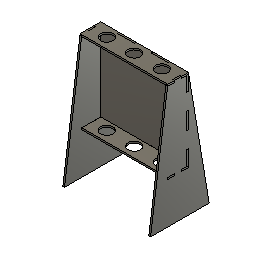
OpenColumnx3_FitSBS_v1 v6 (Autodesk Fusion 360 design; units mm, degrees)
Autodesk Fusion 360 part; units mm, degrees
sketch "Sketch1" plane through (0, 0, 0) normal (0, 1, 0) x (1, 0, 0)
  line L0 (0, 0) -> (127.76, 0)
  line L1 (127.76, 0) -> (127.76, 85.48)
  line L2 (127.76, 85.48) -> (0, 85.48)
  line L3 (0, 85.48) -> (0, 0)
  line L4 (0, 85.48) -> (2.5, 85.48)
  line L5 (2.5, 85.48) -> (2.5, 0)
  line L6 (2.5, 0) -> (0, 0)
  line L7 (0, 0) -> (0, 85.48)
  line L8 (127.76, 85.48) -> (125.26, 85.48)
  line L9 (125.26, 85.48) -> (125.26, 0)
  line L10 (125.26, 0) -> (127.76, 0)
  line L11 (127.76, 0) -> (127.76, 85.48)
  dimension "d1" = 127.76
  dimension "d2" = 85.48
  dimension "d3" = 2.5
  dimension "d4" = 85.48
  dimension "d5" = 2.5
  constraint horizontal L0
  constraint vertical L1
  constraint horizontal L2
  constraint vertical L3
  constraint coincident L0.start L3.end
  constraint horizontal L4
  constraint vertical L5
  constraint horizontal L6
  constraint vertical L7
  constraint horizontal L8
  constraint vertical L9
  constraint horizontal L10
  constraint vertical L11
  constraint coincident L0 L9.end
  measures "d1" distance of L0.start L0.end
  measures "d2" distance of L0.start L2.end
  measures "d3" distance of L2.end L4.end
  measures "d4" distance of L2.end L0.start
  measures "d5" distance of L1.end L8.end
ref_plane "WorkPlane1" through (0, 45, 0) normal (0, 1, 0) x (0, 0, 1)
ref_plane "WorkPlane2" through (0, 60, 0) normal (0, 1, 0) x (0, 0, 1)
sketch "Sketch2" plane through (0, 60, 0) normal (0, 1, 0) x (1, 0, 0)
  line L0 (0, 0) -> (127.76, 0)
  line L1 (127.76, 0) -> (127.76, 85.48)
  line L2 (127.76, 85.48) -> (0, 85.48)
  line L3 (0, 85.48) -> (0, 0)
  line L4 (127.76, 55.24) -> (0, 55.24)
  line L5 (0, 55.24) -> (0, 25.24)
  line L6 (0, 25.24) -> (127.76, 25.24)
  line L7 (127.76, 25.24) -> (127.76, 55.24)
  line L8 (127.76, 55.24) -> (0, 25.24) construction
  line L9 (0, 55.24) -> (127.76, 25.24) construction
  line L10 (0, 25.24) -> (2.5, 25.24)
  line L11 (2.5, 25.24) -> (2.5, 55.24)
  line L12 (2.5, 55.24) -> (0, 55.24)
  line L13 (0, 55.24) -> (0, 25.24)
  line L14 (127.76, 25.24) -> (125.26, 25.24)
  line L15 (125.26, 25.24) -> (125.26, 55.24)
  line L16 (125.26, 55.24) -> (127.76, 55.24)
  line L17 (127.76, 55.24) -> (127.76, 25.24)
  circle A0 centre (63.88, 40.24) radius 9
  circle A1 centre (63.88, 40.24) radius 18
  circle A2 centre (23.88, 40.24) radius 9
  circle A3 centre (23.88, 40.24) radius 18
  circle A4 centre (103.88, 40.24) radius 9
  circle A5 centre (103.88, 40.24) radius 18
  line L18 (127.76, 25.24) -> (125.26, 25.24)
  line L19 (0, 25.24) -> (2.5, 25.24)
  line L20 (0, 25.24) -> (2.5, 25.24)
  line L21 (127.76, 35.24) -> (125.26, 35.24)
  line L22 (0, 35.24) -> (2.5, 35.24)
  line L23 (127.76, 45.24) -> (125.26, 45.24)
  line L24 (0, 45.24) -> (2.5, 45.24)
  line L25 (127.76, 55.24) -> (125.26, 55.24)
  line L26 (0, 55.24) -> (2.5, 55.24)
  line L27 (0, 55.24) -> (127.76, 55.24)
  line L28 (127.76, 55.24) -> (127.76, 52.74)
  line L29 (127.76, 52.74) -> (0, 52.74)
  line L30 (0, 52.74) -> (0, 55.24)
  line L31 (2.5, 55.24) -> (2.5, 52.74)
  line L32 (27.052, 55.24) -> (27.052, 52.74)
  line L33 (51.604, 55.24) -> (51.604, 52.74)
  line L34 (76.156, 55.24) -> (76.156, 52.74)
  line L35 (100.708, 55.24) -> (100.708, 52.74)
  line L36 (125.26, 55.24) -> (125.26, 52.74)
  line L37 (2.5, 52.74) -> (0, 52.74)
  line L38 (0, 52.74) -> (0, 55.24)
  line L39 (0, 55.24) -> (2.5, 55.24)
  line L40 (2.5, 55.24) -> (2.5, 52.74)
  line L41 (125.26, 52.74) -> (127.76, 52.74)
  line L42 (127.76, 52.74) -> (127.76, 55.24)
  line L43 (127.76, 55.24) -> (125.26, 55.24)
  line L44 (125.26, 55.24) -> (125.26, 52.74)
  point P0 (63.88, 40.24)
  dimension "d8" = 127.76
  dimension "d9" = 85.48
  dimension "d10" = 127.76
  dimension "d11" = 30
  dimension "d12" = 2.5
  dimension "d13" = 2.5
  dimension "d14" = 18
  dimension "d15" = 36
  dimension "d18" = 40
  dimension "d19" = 0
  dimension "d33" = 0
  dimension "d34" = 30
  dimension "d37" = 2.5
  dimension "d40" = 122.76
  dimension "d41" = 0
  constraint horizontal L0
  constraint vertical L1
  constraint horizontal L2
  constraint vertical L3
  constraint coincident L0.start L3.end
  constraint horizontal L4
  constraint perpendicular L4 L5
  constraint parallel L4 L6
  constraint parallel L5 L7
  constraint coincident L8 P0
  constraint coincident L9 P0
  constraint horizontal L10
  constraint vertical L11
  constraint horizontal L12
  constraint vertical L13
  constraint coincident L4 L11.end
  constraint horizontal L14
  constraint vertical L15
  constraint horizontal L16
  constraint vertical L17
  constraint coincident L4 L15.end
  constraint coincident P0 A0.centre
  constraint concentric A0 A1
  constraint horizontal L27
  constraint vertical L28
  constraint horizontal L29
  constraint vertical L30
  constraint coincident L29 L31.end
  constraint coincident L11 L31.end
  constraint horizontal L37
  constraint vertical L38
  constraint horizontal L39
  constraint vertical L40
  constraint horizontal L41
  constraint vertical L42
  constraint horizontal L43
  constraint vertical L44
  measures "d8" distance of L0.start L0.end
  measures "d9" distance of L0.start L2.end
  measures "d10" distance of L5.end L6.end
  measures "d11" distance of L4.end L5.end
  measures "d12" distance of L5.end L10.end
  measures "d13" distance of L6.end L14.end
  measures "d14" diameter of A0
  measures "d15" diameter of A1
  measures "d37" distance of L4.end L29.end
extrude "Extrude3" add sketch "Sketch2" along normal blind 2.5 contours L3 L5 L6 L10 L11 L13 L19 L20 L22 | L1 L6 L7 L14 L15 L17 L18 L21 | L6 L11 A3 L29 | L6 L15 A5 L29 | L3 L5 L11 L13 L24 L29 L37 | L6 A3 L29 | L1 L7 L15 L17 L23 L29 L41 | L6 A5 L29 | L3 L4 L5 L11 L12 L13 L26 L27 L29 L30 L31 L37 L38 L39 L40 | L6 A1 A3 L29 | L4 L11 A3 L27 L29 L31 L40 | L4 A3 L27 L29 L32 | L1 L4 L7 L15 L16 L17 L25 L27 L28 L29 L36 L41 L42 L43 L44 | L6 A1 A5 L29 | L6 A1 L29 | L4 L15 A5 L27 L29 L36 L44 | L4 A5 L27 L29 L35 | L4 A1 L27 L33 | L4 A1 L27 L29 L33 L34 | L4 A1 L27 L34 picked at (22.678, 54.4067) picked at (105.082, 54.4067) makes body 1
copy_body "CopyPasteBodies3" bodies 1 makes body 2
move_body "Move3" bodies 2 to x (1, 0, 0) y (0, 1, 0) z (0, 0, 1) at (0, 117.5, 0)
sketch "Sketch4" plane through (0, 180, 0) normal (0, 1, 0) x (-1, 0, 0)
  circle A0 centre (-103.88, -40.24) radius 9
  circle A1 centre (-23.88, -40.24) radius 9
  circle A2 centre (-63.88, -40.24) radius 9
  line L0 (-127.76, -55.24) -> (-100.708, -55.24)
  line L1 (-100.708, -55.24) -> (-100.708, -52.74)
  line L2 (-100.708, -52.74) -> (-76.156, -52.74)
  line L3 (-76.156, -52.74) -> (-76.156, -55.24)
  line L4 (-76.156, -55.24) -> (-51.604, -55.24)
  line L5 (-51.604, -55.24) -> (-51.604, -52.74)
  line L6 (-51.604, -52.74) -> (-27.052, -52.74)
  line L7 (-27.052, -52.74) -> (-27.052, -55.24)
  line L8 (-27.052, -55.24) -> (0, -55.24)
  line L9 (0, -55.24) -> (0, -45.24)
  line L10 (0, -45.24) -> (-2.5, -45.24)
  line L11 (-2.5, -45.24) -> (-2.5, -35.24)
  line L12 (-2.5, -35.24) -> (0, -35.24)
  line L13 (0, -35.24) -> (0, -25.24)
  line L14 (0, -25.24) -> (-127.76, -25.24)
  line L15 (-127.76, -25.24) -> (-127.76, -35.24)
  line L16 (-127.76, -35.24) -> (-125.26, -35.24)
  line L17 (-125.26, -35.24) -> (-125.26, -45.24)
  line L18 (-125.26, -45.24) -> (-127.76, -45.24)
  line L19 (-127.76, -45.24) -> (-127.76, -55.24)
  line L20 (-127.76, -25.24) -> (-125.26, -25.24)
  line L21 (-125.26, -25.24) -> (-125.26, -55.24)
  line L22 (-125.26, -55.24) -> (-127.76, -55.24)
  line L23 (-127.76, -55.24) -> (-127.76, -25.24)
  line L24 (0, -25.24) -> (-2.5, -25.24)
  line L25 (-2.5, -25.24) -> (-2.5, -55.24)
  line L26 (-2.5, -55.24) -> (0, -55.24)
  line L27 (0, -55.24) -> (0, -25.24)
  dimension "d44" = 2.5
  dimension "d45" = 30
  dimension "d46" = 2.5
  dimension "d47" = 30
  constraint horizontal L20
  constraint vertical L21
  constraint horizontal L22
  constraint vertical L23
  constraint coincident L14.end L15.start
  constraint horizontal L24
  constraint vertical L25
  constraint horizontal L26
  constraint vertical L27
  constraint coincident L13.end L14.start
  measures "d44" distance of L14.end L20.end
  measures "d45" distance of L14.end L0.start
  measures "d46" distance of L13.end L24.end
  measures "d47" distance of L13.end L8.end
loft "Loft3" add profiles "Sketch4", "Sketch1" section 1 contours L0 L18 L19 L21 L22 L23 | L16 L17 L18 L21 L23 | L14 L15 L16 L20 L21 L23 section 2 contours L0 L1 L2 L8 L9 L10 L11 separate body makes body 3
loft "Loft4" add profiles "Sketch4", "Sketch1" section 1 contours L12 L13 L14 L24 L25 L27 | L10 L11 L12 L25 L27 | L8 L9 L10 L25 L26 L27 section 2 contours L0 L2 L3 L4 L5 L6 L7 separate body makes body 4
ref_plane "WorkPlane3" through (39.328, 178.75, -52.74) normal (0, 0, -1) x (-1, 0, 0)
extrude "Extrude4" add sketch "Sketch2" along normal blind 120 separate body contours L3 L4 L5 L11 L12 L13 L26 L27 L29 L30 L31 L37 L38 L39 L40 | L4 L11 A3 L27 L29 L31 L40 | L4 A3 L27 L29 L32 | L1 L4 L7 L15 L16 L17 L25 L27 L28 L29 L36 L41 L42 L43 L44 | L4 A3 L27 L29 L32 | L4 L15 A5 L27 L29 L36 L44 | L4 A1 A5 L27 L29 L34 | L4 A5 L27 L29 L35 | L4 A5 L27 L29 L35 | L4 A1 A3 L27 L29 L33 | A1 L29 L33 | A1 L29 L34 | L4 A1 L27 L33 | L4 A1 L27 L29 L33 L34 | L4 A1 L27 L34 makes body 5
sketch "Sketch7" plane through (0, 0, -55.24) normal (0, 0, -1) x (-1, 0, 0)
  line L0 (-127.76, 60) -> (0, 60)
  line L1 (0, 60) -> (0, 180)
  line L2 (0, 180) -> (-127.76, 180)
  line L3 (-127.76, 180) -> (-127.76, 60)
  line L4 (-127.76, 180) -> (0, 180)
  line L5 (0, 180) -> (0, 60)
  line L6 (0, 60) -> (-127.76, 60)
  line L7 (-127.76, 60) -> (-127.76, 180)
  line L8 (-127.76, 180) -> (-125.26, 180)
  line L9 (-125.26, 180) -> (-125.26, 60)
  line L10 (-125.26, 60) -> (-127.76, 60)
  line L11 (-127.76, 60) -> (-127.76, 180)
  line L12 (0, 180) -> (-2.5, 180)
  line L13 (-2.5, 180) -> (-2.5, 60)
  line L14 (-2.5, 60) -> (0, 60)
  line L15 (0, 60) -> (0, 180)
  line L16 (-127.76, 180) -> (-125.26, 180)
  line L17 (0, 180) -> (-2.5, 180)
  line L18 (0, 156) -> (-2.5, 156)
  line L19 (0, 132) -> (-2.5, 132)
  line L20 (0, 108) -> (-2.5, 108)
  line L21 (0, 84) -> (-2.5, 84)
  line L22 (0, 60) -> (-2.5, 60)
  line L23 (-127.76, 156) -> (-125.26, 156)
  line L24 (-127.76, 132) -> (-125.26, 132)
  line L25 (-127.76, 108) -> (-125.26, 108)
  line L26 (-127.76, 84) -> (-125.26, 84)
  line L27 (-127.76, 60) -> (-125.26, 60)
  dimension "d51" = 2.5
  dimension "d52" = 2.5
  dimension "d53" = 120
  dimension "d56" = 0
  dimension "d57" = -120
  dimension "d60" = 0
  dimension "d61" = -120
  constraint horizontal L4
  constraint vertical L5
  constraint horizontal L6
  constraint vertical L7
  constraint coincident L0.end L1.start
  constraint coincident L2.end L3.start
  constraint horizontal L8
  constraint vertical L9
  constraint horizontal L10
  constraint vertical L11
  constraint horizontal L12
  constraint vertical L13
  constraint horizontal L14
  constraint vertical L15
  measures "d51" distance of L2.end L8.end
  measures "d52" distance of L1.end L12.end
  measures "d53" distance of L1.end L0.end
extrude "Extrude5" cut sketch "Sketch7" against normal blind 20 contours L3 L7 L9 L11 L25 L26 | L1 L5 L13 L15 L20 L21 | L3 L7 L9 L11 L23 L24 | L1 L5 L13 L15 L18 L19 bodies 5
combine "Combine1" operation cut target body 5 tool bodies 2 1 keep tools
combine "Combine2" operation cut target body 4 tool bodies 2 5 1 keep tools
combine "Combine3" operation cut target body 3 tool bodies 5 2 1 keep tools
sketch "Sketch8" plane through (127.76, 0, 0) normal (1, 0, 0) x (0, 0, -1)
  line L0 (45.24, 62.5) -> (52.74, 62.5)
  line L1 (52.74, 62.5) -> (52.74, 84)
  line L2 (52.74, 84) -> (55.24, 84)
  line L3 (55.24, 84) -> (55.24, 60)
  line L4 (55.24, 60) -> (45.24, 60)
  line L5 (45.24, 60) -> (45.24, 62.5)
  line L6 (25.24, 60) -> (25.24, 62.5)
  line L7 (25.24, 62.5) -> (35.24, 62.5)
  line L8 (35.24, 62.5) -> (35.24, 60)
  line L9 (35.24, 60) -> (25.24, 60)
  line L10 (25.24, 177.5) -> (25.24, 180)
  line L11 (25.24, 180) -> (0, 0)
  line L12 (0, 0) -> (85.48, 0)
  line L13 (85.48, 0) -> (55.24, 180)
  line L14 (55.24, 180) -> (55.24, 156)
  line L15 (55.24, 156) -> (52.74, 156)
  line L16 (52.74, 156) -> (52.74, 177.5)
  line L17 (52.74, 177.5) -> (45.24, 177.5)
  line L18 (45.24, 177.5) -> (45.24, 180)
  line L19 (45.24, 180) -> (35.24, 180)
  line L20 (35.24, 180) -> (35.24, 177.5)
  line L21 (35.24, 177.5) -> (25.24, 177.5)
  line L22 (55.24, 132) -> (55.24, 108)
  line L23 (55.24, 108) -> (52.74, 108)
  line L24 (52.74, 108) -> (52.74, 132)
  line L25 (52.74, 132) -> (55.24, 132)
sketch "Sketch9" plane through (0, 0, -52.74) normal (0, 0, 1) x (1, 0, 0)
  line L0 (0, 62.5) -> (27.052, 62.5)
  line L1 (27.052, 62.5) -> (27.052, 60)
  line L2 (27.052, 60) -> (51.604, 60)
  line L3 (51.604, 60) -> (51.604, 62.5)
  line L4 (51.604, 62.5) -> (76.156, 62.5)
  line L5 (76.156, 62.5) -> (76.156, 60)
  line L6 (76.156, 60) -> (100.708, 60)
  line L7 (100.708, 60) -> (100.708, 62.5)
  line L8 (100.708, 62.5) -> (127.76, 62.5)
  line L9 (127.76, 62.5) -> (127.76, 84)
  line L10 (127.76, 84) -> (125.26, 84)
  line L11 (125.26, 84) -> (125.26, 108)
  line L12 (125.26, 108) -> (127.76, 108)
  line L13 (127.76, 108) -> (127.76, 132)
  line L14 (127.76, 132) -> (125.26, 132)
  line L15 (125.26, 132) -> (125.26, 156)
  line L16 (125.26, 156) -> (127.76, 156)
  line L17 (127.76, 156) -> (127.76, 177.5)
  line L18 (127.76, 177.5) -> (100.708, 177.5)
  line L19 (100.708, 177.5) -> (100.708, 180)
  line L20 (100.708, 180) -> (76.156, 180)
  line L21 (76.156, 180) -> (76.156, 177.5)
  line L22 (76.156, 177.5) -> (51.604, 177.5)
  line L23 (51.604, 177.5) -> (51.604, 180)
  line L24 (51.604, 180) -> (27.052, 180)
  line L25 (27.052, 180) -> (27.052, 177.5)
  line L26 (27.052, 177.5) -> (0, 177.5)
  line L27 (0, 177.5) -> (0, 156)
  line L28 (0, 156) -> (2.5, 156)
  line L29 (2.5, 156) -> (2.5, 132)
  line L30 (2.5, 132) -> (0, 132)
  line L31 (0, 132) -> (0, 108)
  line L32 (0, 108) -> (2.5, 108)
  line L33 (2.5, 108) -> (2.5, 84)
  line L34 (2.5, 84) -> (0, 84)
  line L35 (0, 84) -> (0, 62.5)
sketch "Sketch10" plane through (0, 180, 0) normal (0, 1, 0) x (-1, 0, 0)
  circle A0 centre (-103.88, -40.24) radius 9
  circle A1 centre (-23.88, -40.24) radius 9
  circle A2 centre (-63.88, -40.24) radius 9
  line L0 (-127.76, -55.24) -> (-100.708, -55.24)
  line L1 (-100.708, -55.24) -> (-100.708, -52.74)
  line L2 (-100.708, -52.74) -> (-76.156, -52.74)
  line L3 (-76.156, -52.74) -> (-76.156, -55.24)
  line L4 (-76.156, -55.24) -> (-51.604, -55.24)
  line L5 (-51.604, -55.24) -> (-51.604, -52.74)
  line L6 (-51.604, -52.74) -> (-27.052, -52.74)
  line L7 (-27.052, -52.74) -> (-27.052, -55.24)
  line L8 (-27.052, -55.24) -> (0, -55.24)
  line L9 (0, -55.24) -> (0, -45.24)
  line L10 (0, -45.24) -> (-2.5, -45.24)
  line L11 (-2.5, -45.24) -> (-2.5, -35.24)
  line L12 (-2.5, -35.24) -> (0, -35.24)
  line L13 (0, -35.24) -> (0, -25.24)
  line L14 (0, -25.24) -> (-127.76, -25.24)
  line L15 (-127.76, -25.24) -> (-127.76, -35.24)
  line L16 (-127.76, -35.24) -> (-125.26, -35.24)
  line L17 (-125.26, -35.24) -> (-125.26, -45.24)
  line L18 (-125.26, -45.24) -> (-127.76, -45.24)
  line L19 (-127.76, -45.24) -> (-127.76, -55.24)
sketch "Sketch11" plane through (0, 0, 0) normal (-1, 0, 0) x (0, 0, 1)
  line L0 (-55.24, 60) -> (-55.24, 84)
  line L1 (-55.24, 84) -> (-52.74, 84)
  line L2 (-52.74, 84) -> (-52.74, 62.5)
  line L3 (-52.74, 62.5) -> (-45.24, 62.5)
  line L4 (-45.24, 62.5) -> (-45.24, 60)
  line L5 (-45.24, 60) -> (-55.24, 60)
  line L6 (-35.24, 60) -> (-35.24, 62.5)
  line L7 (-35.24, 62.5) -> (-25.24, 62.5)
  line L8 (-25.24, 62.5) -> (-25.24, 60)
  line L9 (-25.24, 60) -> (-35.24, 60)
  line L10 (-52.74, 177.5) -> (-52.74, 156)
  line L11 (-52.74, 156) -> (-55.24, 156)
  line L12 (-55.24, 156) -> (-55.24, 180)
  line L13 (-55.24, 180) -> (-85.48, 0)
  line L14 (-85.48, 0) -> (0, 0)
  line L15 (0, 0) -> (-25.24, 180)
  line L16 (-25.24, 180) -> (-25.24, 177.5)
  line L17 (-25.24, 177.5) -> (-35.24, 177.5)
  line L18 (-35.24, 177.5) -> (-35.24, 180)
  line L19 (-35.24, 180) -> (-45.24, 180)
  line L20 (-45.24, 180) -> (-45.24, 177.5)
  line L21 (-45.24, 177.5) -> (-52.74, 177.5)
  line L22 (-55.24, 108) -> (-55.24, 132)
  line L23 (-55.24, 132) -> (-52.74, 132)
  line L24 (-52.74, 132) -> (-52.74, 108)
  line L25 (-52.74, 108) -> (-55.24, 108)
sketch "Sketch12" plane through (0, 62.5, 0) normal (0, 1, 0) x (-1, 0, 0)
  circle A0 centre (-103.88, -40.24) radius 9
  circle A1 centre (-23.88, -40.24) radius 9
  circle A2 centre (-63.88, -40.24) radius 9
  line L0 (-127.76, -55.24) -> (-100.708, -55.24)
  line L1 (-100.708, -55.24) -> (-100.708, -52.74)
  line L2 (-100.708, -52.74) -> (-76.156, -52.74)
  line L3 (-76.156, -52.74) -> (-76.156, -55.24)
  line L4 (-76.156, -55.24) -> (-51.604, -55.24)
  line L5 (-51.604, -55.24) -> (-51.604, -52.74)
  line L6 (-51.604, -52.74) -> (-27.052, -52.74)
  line L7 (-27.052, -52.74) -> (-27.052, -55.24)
  line L8 (-27.052, -55.24) -> (0, -55.24)
  line L9 (0, -55.24) -> (0, -45.24)
  line L10 (0, -45.24) -> (-2.5, -45.24)
  line L11 (-2.5, -45.24) -> (-2.5, -35.24)
  line L12 (-2.5, -35.24) -> (0, -35.24)
  line L13 (0, -35.24) -> (0, -25.24)
  line L14 (0, -25.24) -> (-127.76, -25.24)
  line L15 (-127.76, -25.24) -> (-127.76, -35.24)
  line L16 (-127.76, -35.24) -> (-125.26, -35.24)
  line L17 (-125.26, -35.24) -> (-125.26, -45.24)
  line L18 (-125.26, -45.24) -> (-127.76, -45.24)
  line L19 (-127.76, -45.24) -> (-127.76, -55.24)
